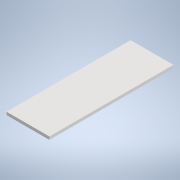
# Autodesk Inventor part: Arm Rest
Saved by Autodesk Inventor 2021.1 (Build 251245000, 245)
## iProperties
Created: 2020-08-02
Part Number: Arm Rest
Material: Generic
Document SubType Name: Modeling
Designer: adick
Density: 1 g/cm^3
Appearance: Default
Author: adick
Autodesk Inventor part; units mm, degrees
ref_plane "YZ Plane" through (0, 0, 0) normal (1, 0, 0) x (0, 1, 0)
ref_plane "XZ Plane" through (0, 0, 0) normal (0, 1, 0) x (-1, 0, 0)
ref_plane "XY Plane" through (0, 0, 0) normal (0, 0, 1) x (1, 0, 0)
sketch "Sketch1" plane through (0, 0, 0) normal (0, 0, 1) x (1, 0, 0)
  line L0 (-135, -7) -> (-35.423, -7) projected
  line L1 (-128.65, -70.65) -> (-128.65, -7) projected
  line L2 (135, -70.65) -> (-135, -70.65) projected
  line L3 (-128.65, -7) -> (-35.423, -7)
  line L4 (-35.423, -7) -> (-35.423, -13.3614)
  line L5 (-35.423, -13.3614) -> (-128.65, -13.3614)
  line L6 (-128.65, -13.3614) -> (-128.65, -7)
  point P0 (0, 0)
  constraints: 8 end point, 2 parallel, 1 horizontal, 1 perpendicular
extrude "Extrusion1" add sketch "Sketch1" along normal blind 270
body "Solid1"
